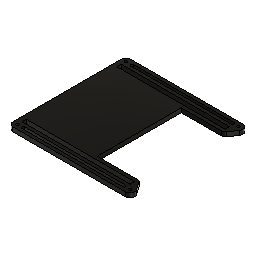
AssemblyCameraHolder v6 (Autodesk Fusion 360 archive; units mm, degrees)
design "CameraBase"
Autodesk Fusion 360 part; units mm, degrees
sketch "Sketch1" plane through (0, 0, 0) normal (0, 0, 1) x (1, 0, 0)
  line L0 (-62.5, 60.2) -> (62.5, 60.2) construction
  line L1 (62.5, 60.2) -> (62.5, -60.2) construction
  line L2 (62.5, -60.2) -> (-62.5, -60.2) construction
  line L3 (-62.5, -60.2) -> (-62.5, 60.2) construction
  line L4 (0, 0) -> (0, 60.2) construction
  line L5 (0, 0) -> (-62.5, 0) construction
  circle A0 centre (62.5, 60.2) radius 1.5
  circle A1 centre (-62.5, 60.2) radius 1.5
  circle A2 centre (62.5, -60.2) radius 1.5
  circle A3 centre (-62.5, -60.2) radius 1.5
  line L6 (-62.5, -65.2) -> (62.5, -65.2)
  line L7 (-67.5, -60.2) -> (-67.5, 60.2)
  line L8 (-62.5, 65.2) -> (62.5, 65.2)
  line L9 (-56, 61.7) -> (56, 61.7)
  line L10 (-56, 58.7) -> (56, 58.7)
  arc A4 (-56, 61.7) -> (-56, 58.7) centre (-56, 60.2) ccw
  arc A5 (56, 58.7) -> (56, 61.7) centre (56, 60.2) ccw
  arc A6 (-67.5, 60.2) -> (-62.5, 65.2) centre (-62.5, 60.2) ccw construction
  arc A7 (-62.5, 65.2) -> (-67.5, 60.2) centre (-62.5, 60.2) ccw
  line L11 (-62.5, 55.2) -> (57.5, 55.2)
  line L12 (57.5, 55.2) -> (57.5, 50.4)
  line L13 (57.5, 50.4) -> (-62.5, 50.4)
  line L14 (-62.5, 50.4) -> (-62.5, 55.2)
  line L15 (66.6668, 57.4363) -> (60.6251, 48.3272)
  arc A8 (62.5, 65.2) -> (66.6668, 57.4363) centre (62.5, 60.2) ccw construction
  arc A9 (66.6668, 57.4363) -> (62.5, 65.2) centre (62.5, 60.2) ccw
  arc A10 (60.6251, 48.3272) -> (60.6251, 48.3272) centre (57.5, 50.4) ccw construction
  line L16 (-56, -58.7) -> (56, -58.7)
  line L17 (-56, -61.7) -> (56, -61.7)
  arc A11 (-56, -58.7) -> (-56, -61.7) centre (-56, -60.2) ccw
  arc A12 (56, -61.7) -> (56, -58.7) centre (56, -60.2) ccw
  line L18 (-62.5, -55.2) -> (57.5, -55.2)
  line L19 (57.5, -55.2) -> (57.5, -50.4)
  line L20 (57.5, -50.4) -> (-62.5, -50.4)
  line L21 (-62.5, -50.4) -> (-62.5, -55.2)
  line L22 (57.5, -60.2) -> (57.5, -55.2) construction
  line L23 (60.6251, -48.3272) -> (66.6668, -57.4363)
  line L24 (57.5, -46.65) -> (12.5, -46.65)
  line L25 (12.5, 46.65) -> (12.5, -46.65)
  arc A13 (57.5, -46.65) -> (60.6251, -48.3272) centre (57.5, -50.4) ccw construction
  arc A14 (60.6251, -48.3272) -> (57.5, -46.65) centre (57.5, -50.4) ccw
  arc A15 (66.6668, -57.4363) -> (62.5, -65.2) centre (62.5, -60.2) ccw construction
  arc A16 (62.5, -65.2) -> (66.6668, -57.4363) centre (62.5, -60.2) ccw
  arc A17 (-62.5, -65.2) -> (-67.5, -60.2) centre (-62.5, -60.2) ccw construction
  arc A18 (-67.5, -60.2) -> (-62.5, -65.2) centre (-62.5, -60.2) ccw
  line L26 (57.5, -50.4) -> (57.5, 50.4) construction
  line L27 (57.5, 46.65) -> (12.5, 46.65)
  arc A19 (60.6251, 48.3272) -> (57.5, 46.65) centre (57.5, 50.4) ccw construction
  arc A20 (57.5, 46.65) -> (60.6251, 48.3272) centre (57.5, 50.4) ccw
  line L28 (57.5, 55.2) -> (57.5, 60.2) construction
  point P0 (-62.5, 0)
  point P1 (0, 60.2)
  dimension "d1" = 125
  dimension "d2" = 120.4
  dimension "d3" = 3
  dimension "d4" = 3
  dimension "d5" = 3
  dimension "d6" = 3
  dimension "d7" = 10
  dimension "d8" = 10
  dimension "d9" = 10
  dimension "d10" = 10
  dimension "d11" = 3
  dimension "d12" = 5
  dimension "d13" = 6.5
  dimension "d14" = 6.5
  dimension "d16" = 4.8
  dimension "d17" = 5
  dimension "d19" = 3
  dimension "d20" = 5
  dimension "d21" = 6.5
  dimension "d22" = 6.5
  dimension "d23" = 4.8
  dimension "d24" = 7.5
  dimension "d25" = 50
  dimension "d28" = 3.75
  constraint horizontal L0
  constraint vertical L1
  constraint horizontal L2
  constraint vertical L3
  constraint midpoint L3 P0
  constraint midpoint L0 P1
  constraint coincident L4.start L5.start
  constraint coincident P1 L4.end
  constraint coincident P0 L5.end
  constraint vertical L4
  constraint horizontal L5
  constraint coincident L0.end L1.start
  constraint coincident L0.start L3.end
  constraint coincident L1.end L2.start
  constraint coincident L2.end L3.start
  constraint concentric A1 A6
  constraint concentric A0 A8
  constraint concentric A2 A15
  constraint concentric A3 A17
  constraint tangent L6 A15
  constraint perpendicular L1 L6
  constraint tangent L7 A6
  constraint perpendicular L6 L7
  constraint tangent L8 A8
  constraint perpendicular L7 L8
  constraint parallel L8 L9
  constraint parallel L0 L10
  constraint tangent L10 A4
  constraint tangent L9 A4
  constraint tangent L10 A5
  constraint tangent L9 A5
  constraint concentric A6 A7
  constraint horizontal L11
  constraint vertical L12
  constraint horizontal L13
  constraint vertical L14
  constraint coincident L3 L11.start
  constraint coincident L12.end L13.start
  constraint tangent L15 A10
  constraint tangent L15 A8
  constraint perpendicular L2 L25
  constraint concentric A8 A9
  constraint perpendicular L3 L16
  constraint parallel L16 L17
  constraint tangent L16 A11
  constraint tangent L17 A11
  constraint tangent L16 A12
  constraint tangent L17 A12
  constraint horizontal L18
  constraint vertical L19
  constraint horizontal L20
  constraint vertical L21
  constraint coincident L3 L18.start
  constraint midpoint A12 L22.start
  constraint tangent L22 A15
  constraint coincident L19.end L20.start
  constraint tangent L23 A15
  constraint tangent L23 A13
  constraint tangent L24 A13
  constraint perpendicular L24 L25
  constraint concentric A13 A14
  constraint concentric A15 A16
  constraint coincident L18.start A17
  constraint concentric A17 A18
  constraint vertical L26
  constraint coincident L26 L27.start
  constraint tangent A10 L27
  constraint tangent L15 A19
  constraint concentric A19 A20
  constraint collinear L12 L26
  constraint midpoint A5 L28.end
  constraint collinear L12 L28
  measures "d1" distance of L0.start L0.end
  measures "d2" distance of L0.start L2.end
  measures "d3" diameter of A0
  measures "d4" diameter of A1
  measures "d5" diameter of A2
  measures "d6" diameter of A3
  measures "d7" diameter of A6
  measures "d8" diameter of A8
  measures "d9" diameter of A15
  measures "d10" diameter of A17
  measures "d11" distance of L9 L10
  measures "d12" distance of L8 A4.centre
  measures "d13" distance of L0.start A4.centre
  measures "d14" distance of L0.end A5.centre
  measures "d16" distance of L11.start L13.end
  measures "d17" distance of L0 L11
  measures "d19" distance of L16 L17
  measures "d20" distance of L6 A11.centre
  measures "d21" distance of L2.end A11.centre
  measures "d22" distance of L1.end A12.centre
  measures "d23" distance of L18.start L20.end
  measures "d24" diameter of A13
  measures "d25" distance of L1 L25
  measures "d28" radius of A19
extrude "Extrude1" add sketch "Sketch1" along normal blind 4.8

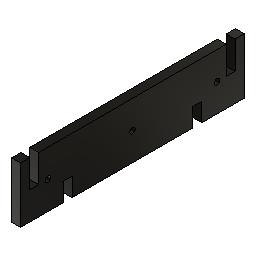
design "CameraHolder"
Autodesk Fusion 360 part; units mm, degrees
sketch "Sketch1" plane through (0, 0, 0) normal (1, 0, 0) x (0, 1, 0)
  line L0 (-60.2, 30) -> (-60.2, 0)
  line L1 (-60.2, 0) -> (-37.3, 0)
  line L2 (-37.3, 0) -> (-37.3, 10)
  line L3 (-37.3, 10) -> (-32.5, 10)
  line L4 (-32.5, 10) -> (-32.5, 0)
  line L5 (-32.5, 0) -> (32.5, 0)
  line L6 (32.5, 0) -> (32.5, 10)
  line L7 (32.5, 10) -> (37.3, 10)
  line L8 (37.3, 10) -> (37.3, 0)
  line L9 (37.3, 0) -> (60.2, 0)
  line L10 (60.2, 0) -> (60.2, 30)
  line L11 (60.2, 30) -> (55.2, 30)
  line L12 (55.2, 30) -> (55.2, 15)
  line L13 (55.2, 15) -> (50.4, 15)
  line L14 (50.4, 15) -> (50.4, 30)
  line L15 (50.4, 30) -> (-50.4, 30)
  line L16 (-50.4, 30) -> (-50.4, 15)
  line L17 (-50.4, 15) -> (-55.2, 15)
  line L18 (-55.2, 15) -> (-55.2, 30)
  line L19 (-55.2, 30) -> (-60.2, 30)
  line L20 (-55.2, 30) -> (-50.4, 30) construction
  line L21 (50.4, 30) -> (55.2, 30) construction
  line L22 (37.3, 0) -> (32.5, 0) construction
  line L23 (-32.5, 0) -> (-37.3, 0) construction
  line L24 (-50.4, 15) -> (50.4, 15) construction
  line L25 (0, 0) -> (0, 15) construction
  line L26 (0, 15) -> (0, 30) construction
  circle A0 centre (0, 15) radius 1.5
  circle A1 centre (-45.4, 15) radius 1.5
  circle A2 centre (45.4, 15) radius 1.5
  line L27 (-32.5, 10) -> (32.5, 10) construction
  point P0 (0, 15)
  point P1 (0, 15)
  point P2 (0, 30)
  dimension "d1" = 4.8
  dimension "d2" = 4.8
  dimension "d3" = 4.8
  dimension "d4" = 4.8
  dimension "d7" = 15
  dimension "d9" = 30
  dimension "d10" = 65
  dimension "d11" = 120.4
  dimension "d12" = 100.8
  dimension "d13" = 5
  dimension "d14" = 3
  dimension "d15" = 3
  dimension "d16" = 5
  dimension "d17" = 3
  dimension "d18" = 5
  dimension "d21" = 10
  constraint vertical L0
  constraint perpendicular L0 L1
  constraint perpendicular L1 L2
  constraint perpendicular L0 L3
  constraint perpendicular L1 L4
  constraint perpendicular L4 L5
  constraint perpendicular L3 L6
  constraint perpendicular L6 L7
  constraint perpendicular L7 L8
  constraint perpendicular L8 L9
  constraint perpendicular L9 L10
  constraint perpendicular L0 L11
  constraint perpendicular L11 L12
  constraint perpendicular L0 L13
  constraint perpendicular L13 L14
  constraint perpendicular L14 L15
  constraint perpendicular L15 L16
  constraint perpendicular L16 L17
  constraint perpendicular L15 L18
  constraint perpendicular L0 L19
  constraint perpendicular L18 L20
  constraint perpendicular L12 L21
  constraint perpendicular L6 L22
  constraint perpendicular L2 L23
  constraint perpendicular L14 L24
  constraint midpoint L24 P1
  constraint midpoint L5 L25.start
  constraint midpoint L15 P2
  constraint coincident L25.start origin
  constraint coincident P1 P0
  constraint coincident P2 L26.end
  constraint coincident L24 A1.centre
  constraint coincident L24 A2.centre
  constraint perpendicular L24 L25
  constraint perpendicular L6 L27
  measures "d1" distance of L2 L4
  measures "d2" distance of L6 L8
  measures "d3" distance of L12 L14
  measures "d4" distance of L16 L18
  measures "d7" distance of L15 L24
  measures "d9" distance of L0.start L0.end
  measures "d10" distance of L4 L6
  measures "d11" distance of L0 L10
  measures "d12" distance of L14 L16
  measures "d13" distance of L10 L12
  measures "d14" diameter of A0
  measures "d15" diameter of A1
  measures "d16" distance of L16 A1.centre
  measures "d17" diameter of A2
  measures "d18" distance of L14 A2.centre
  measures "d21" distance of L3 L5
extrude "Extrude1" add sketch "Sketch1" along normal blind 4.8

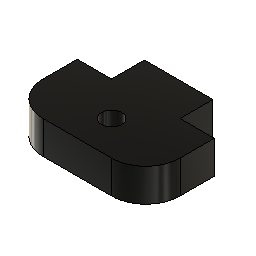
design "ThrowerLock"
Autodesk Fusion 360 part; units mm, degrees
sketch "Sketch1" plane through (0, 0, 0) normal (0, 0, 1) x (1, 0, 0)
  line L0 (-5, 9.8) -> (5, 9.8)
  line L1 (5, 9.8) -> (5, 5)
  line L2 (5, 5) -> (10, 5)
  line L3 (10, 5) -> (10, 0)
  line L4 (5, -5) -> (-5, -5)
  line L5 (-10, 0) -> (-10, 5)
  line L6 (-10, 5) -> (-5, 5)
  line L7 (-5, 5) -> (-5, 9.8)
  line L8 (0, 0) -> (0, 9.8) construction
  line L9 (0, 0) -> (10, 0) construction
  line L10 (0, 0) -> (0, -5) construction
  line L11 (-5, 5) -> (-5, 0) construction
  line L12 (0, 0) -> (-5, 0) construction
  circle A0 centre (0, 0) radius 1.5
  line L13 (-10, -5) -> (-10, 0) construction
  line L14 (-5, -5) -> (-10, -5) construction
  arc A1 (-5, -5) -> (-10, 0) centre (-5, 0) ccw construction
  arc A2 (-10, 0) -> (-5, -5) centre (-5, 0) ccw
  line L15 (10, -5) -> (5, -5) construction
  line L16 (10, 0) -> (10, -5) construction
  arc A3 (10, 0) -> (5, -5) centre (5, 0) ccw construction
  arc A4 (5, -5) -> (10, 0) centre (5, 0) ccw
  point P0 (0, 9.8)
  point P1 (0, -5)
  point P2 (5, 0)
  dimension "d1" = 10
  dimension "d2" = 5
  dimension "d3" = 4.8
  dimension "d5" = 3
  dimension "d6" = 10
  constraint horizontal L0
  constraint perpendicular L0 L1
  constraint perpendicular L1 L2
  constraint perpendicular L2 L3
  constraint perpendicular L1 L4
  constraint perpendicular L4 L5
  constraint perpendicular L5 L6
  constraint vertical L7
  constraint collinear L2 L6
  constraint midpoint L0 P0
  constraint coincident L8.start L9.start
  constraint coincident L0 P0
  constraint perpendicular L0 L8
  constraint coincident L3 L9.end
  constraint perpendicular L3 L9
  constraint coincident P0 L8.end
  constraint coincident L3.end L9.end
  constraint coincident L4 P1
  constraint perpendicular L4 L10
  constraint coincident P1 L10.end
  constraint perpendicular L6 L11
  constraint perpendicular L11 L12
  constraint coincident L11.end L12.end
  constraint tangent L4 A1
  constraint midpoint L9 P2
  constraint coincident P2 A3.centre
  constraint tangent L4 A3
  constraint perpendicular L4 L13
  constraint perpendicular L1 L14
  constraint tangent L14 A3
  constraint concentric A1 A2
  constraint perpendicular L1 L15
  constraint concentric A3 A4
  constraint parallel L3 L16
  constraint tangent L13 A2
  measures "d1" distance of L0.start L0.end
  measures "d2" distance of L1.end L2.end
  measures "d3" distance of L0.start L6.end
  measures "d5" diameter of A0
  measures "d6" distance of L4 L6
extrude "Extrude1" add sketch "Sketch1" along normal blind 4.8

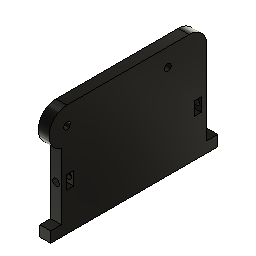
design "CameraHeadHolder"
Autodesk Fusion 360 part; units mm, degrees
sketch "Sketch1" plane through (0, 0, 0) normal (1, 0, 0) x (0, 1, 0)
  line L0 (-32.5, 4.8) -> (-37.3, 4.8)
  line L1 (-37.3, 4.8) -> (-37.3, 0)
  line L2 (-37.3, 0) -> (37.3, 0)
  line L3 (37.3, 0) -> (37.3, 4.8)
  line L4 (37.3, 4.8) -> (32.5, 4.8)
  line L5 (-32.5, 4.8) -> (-32.5, 34.2007)
  line L6 (-30, 49.8) -> (24.5, 49.8)
  line L7 (32.5, 41.8) -> (32.5, 4.8)
  line L8 (-30, 41.8) -> (15, 41.8) construction
  circle A0 centre (-30, 41.8) radius 1.5
  line L9 (15, 41.8) -> (24.5, 41.8) construction
  arc A1 (24.5, 49.8) -> (32.5, 41.8) centre (24.5, 41.8) ccw construction
  arc A2 (32.5, 41.8) -> (24.5, 49.8) centre (24.5, 41.8) ccw
  line L10 (24.5, 49.8) -> (32.5, 49.8) construction
  line L11 (32.5, 49.8) -> (32.5, 41.8) construction
  circle A3 centre (15, 41.8) radius 1.5
  circle A4 centre (-25, 41.8) radius 5 construction
  circle A5 centre (25, 41.8) radius 5 construction
  line L12 (-25, 41.8) -> (25, 41.8) construction
  line L13 (0, 41.8) -> (0, 0) construction
  arc A6 (-32.5, 34.2007) -> (-30, 49.8) centre (-30, 41.8) ccw construction
  arc A7 (-30, 49.8) -> (-32.5, 34.2007) centre (-30, 41.8) ccw
  point P0 (0, 41.8)
  dimension "d1" = 4.8
  dimension "d2" = 4.8
  dimension "d3" = 74.6
  dimension "d4" = 4.8
  dimension "d5" = 4.8
  dimension "d6" = 45
  dimension "d8" = 45
  dimension "d9" = 8
  dimension "d11" = 3
  dimension "d12" = 16
  dimension "d13" = 3
  dimension "d14" = 10
  dimension "d15" = 10
  dimension "d16" = 50
  dimension "d17" = 10
  constraint horizontal L0
  constraint perpendicular L0 L1
  constraint perpendicular L1 L2
  constraint perpendicular L2 L3
  constraint perpendicular L3 L4
  constraint midpoint L2 L13.end
  constraint coincident L13.end origin
  constraint perpendicular L0 L5
  constraint perpendicular L5 L6
  constraint perpendicular L4 L7
  constraint perpendicular L7 L8
  constraint tangent L7 A1
  constraint coincident L9.end A1.centre
  constraint parallel L8 L9
  constraint concentric A1 A2
  constraint perpendicular L5 L10
  constraint perpendicular L4 L11
  constraint coincident L8.end L9.start
  constraint coincident L8 A4.centre
  constraint coincident L9 A5.centre
  constraint coincident A4.centre L12.start
  constraint coincident A5.centre L12.end
  constraint midpoint L12 P0
  constraint coincident P0 L13.start
  constraint vertical L13
  constraint coincident L8.start A0.centre
  constraint tangent L6 A6
  constraint concentric A6 A7
  constraint concentric A0 A7
  measures "d1" distance of L0.start L0.end
  measures "d2" distance of L0.end L1.end
  measures "d3" distance of L1.end L2.end
  measures "d4" distance of L2.end L3.end
  measures "d5" distance of L3.end L4.end
  measures "d6" distance of L4 L6
  measures "d8" distance of L8.start L8.end
  measures "d9" distance of L6 L8
  measures "d11" diameter of A0
  measures "d12" diameter of A1
  measures "d13" diameter of A3
  measures "d14" diameter of A4
  measures "d15" diameter of A5 L6
  measures "d16" distance of A4.centre A5.centre
  measures "d17" distance of L8.end A5.centre
extrude "Extrude1" add sketch "Sketch1" along normal blind 4.8
sketch "Sketch2" plane through (0, -32.5, 0) normal (0, -1, 0) x (1, 0, 0)
  line L0 (0, 34.2007) -> (0, 4.8)
  line L1 (0, 4.8) -> (4.8, 4.8)
  line L2 (4.8, 4.8) -> (4.8, 34.2007)
  line L3 (4.8, 34.2007) -> (0, 34.2007)
  line L4 (0, 4.8) -> (0, 0)
  line L5 (0, 0) -> (4.8, 0)
  line L6 (4.8, 0) -> (4.8, 4.8)
  line L7 (4.8, 4.8) -> (0, 4.8)
  circle A0 centre (2.4, 20) radius 1.5
  dimension "d20" = 3
  dimension "d21" = 20
  dimension "d22" = 2.4
  measures "d20" diameter of A0
  measures "d21" distance of L5 A0.centre
  measures "d22" distance of L2 A0.centre
hole "Hole1" at (2.4, -32.5, 20) direction (0, 1, 0) diameter 3 depth 7.2 tip angle 118
sketch "Sketch3" plane through (0, 32.5, 0) normal (0, 1, 0) x (-1, 0, 0)
  line L0 (0, 4.8) -> (0, 41.8)
  line L1 (0, 41.8) -> (-4.8, 41.8)
  line L2 (-4.8, 41.8) -> (-4.8, 4.8)
  line L3 (-4.8, 4.8) -> (0, 4.8)
  line L4 (0, 0) -> (0, 4.8)
  line L5 (0, 4.8) -> (-4.8, 4.8)
  line L6 (-4.8, 4.8) -> (-4.8, 0)
  line L7 (-4.8, 0) -> (0, 0)
  circle A0 centre (-2.4, 20) radius 1.5
  dimension "d26" = 3
  dimension "d27" = 20
  dimension "d28" = 2.4
  measures "d26" diameter of A0
  measures "d27" distance of L7 A0.centre
  measures "d28" distance of L0 A0.centre
hole "Hole2" at (2.4, 32.5, 20) direction (0, -1, 0) diameter 3 depth 7.2 tip angle 118
sketch "Sketch4" plane through (4.8, 0, 0) normal (1, 0, 0) x (0, 1, 0)
  circle A0 centre (15, 41.8) radius 1.5
  circle A1 centre (-30, 41.8) radius 1.5
  arc A2 (32.5, 41.8) -> (24.5, 49.8) centre (24.5, 41.8) ccw
  line L0 (24.5, 49.8) -> (-30, 49.8)
  arc A3 (-30, 49.8) -> (-32.5, 34.2007) centre (-30, 41.8) ccw
  line L1 (-32.5, 34.2007) -> (-32.5, 4.8)
  line L2 (-32.5, 4.8) -> (-37.3, 4.8)
  line L3 (-37.3, 4.8) -> (-37.3, 0)
  line L4 (-37.3, 0) -> (37.3, 0)
  line L5 (37.3, 0) -> (37.3, 4.8)
  line L6 (37.3, 4.8) -> (32.5, 4.8)
  line L7 (32.5, 4.8) -> (32.5, 41.8)
  line L8 (-32.5, 18.5) -> (-25.3, 18.5) construction
  line L9 (-25.3, 18.5) -> (-25.3, 21.5) construction
  line L10 (-25.3, 21.5) -> (-32.5, 21.5) construction
  line L11 (32.5, 21.5) -> (25.3, 21.5) construction
  line L12 (25.3, 21.5) -> (25.3, 18.5) construction
  line L13 (25.3, 18.5) -> (32.5, 18.5) construction
  line L14 (-25.3, 20) -> (25.3, 20) construction
  line L15 (-30, 17) -> (-27, 17)
  line L16 (-27, 17) -> (-27, 23)
  line L17 (-27, 23) -> (-30, 23)
  line L18 (-30, 23) -> (-30, 17)
  line L19 (-25.3, 20) -> (-27, 20) construction
  line L20 (27, 23) -> (30, 23)
  line L21 (30, 23) -> (30, 17)
  line L22 (30, 17) -> (27, 17)
  line L23 (27, 17) -> (27, 23)
  line L24 (27, 20) -> (25.3, 20) construction
  point P0 (-25.3, 20)
  point P1 (25.3, 20)
  point P2 (-27, 20)
  point P3 (27, 20)
  dimension "d32" = 7.2
  dimension "d33" = 3
  dimension "d34" = 7.2
  dimension "d35" = 3
  dimension "d36" = 20
  dimension "d37" = 3
  dimension "d38" = 6
  dimension "d39" = 2.5
  dimension "d40" = 3
  dimension "d41" = 6
  dimension "d42" = 2.5
  constraint coincident L1 L8.start
  constraint perpendicular L1 L8
  constraint perpendicular L8 L9
  constraint coincident L1 L10.end
  constraint perpendicular L1 L10
  constraint midpoint L9 P0
  constraint coincident L7 L11.start
  constraint perpendicular L7 L11
  constraint perpendicular L11 L12
  constraint coincident L7 L13.end
  constraint perpendicular L7 L13
  constraint midpoint L12 P1
  constraint coincident P0 L14.start
  constraint coincident P1 L14.end
  constraint horizontal L14
  constraint horizontal L15
  constraint vertical L16
  constraint horizontal L17
  constraint vertical L18
  constraint midpoint L16 P2
  constraint coincident P2 L19.end
  constraint horizontal L19
  constraint horizontal L20
  constraint vertical L21
  constraint horizontal L22
  constraint vertical L23
  constraint midpoint L23 P3
  constraint coincident P3 L24.start
  constraint horizontal L24
  measures "d32" distance of L8.start L8.end
  measures "d33" distance of L8.end L9.end
  measures "d34" distance of L11.start L11.end
  measures "d35" distance of L11.end L12.end
  measures "d36" distance of L4 L14
  measures "d37" distance of L15.start L15.end
  measures "d38" distance of L15.start L17.end
  measures "d39" distance of L1 L18
  measures "d40" distance of L20.start L20.end
  measures "d41" distance of L20.start L22.end
  measures "d42" distance of L7 L21
extrude "Extrude2" cut sketch "Sketch4" against normal through all contours L15 L16 L17 L18 | L20 L21 L22 L23

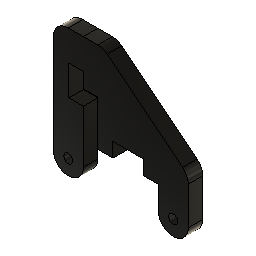
design "CameraHolderSide"
Autodesk Fusion 360 part; units mm, degrees
sketch "Sketch1" plane through (0, 0, 0) normal (0, 1, 0) x (1, 0, 0)
  line L0 (-4.8, 0) -> (-4.8, -10)
  line L1 (0, 0) -> (0, -15)
  line L2 (0, -15) -> (-4.8, -15)
  line L3 (0, 0) -> (-4.8, 0) construction
  line L4 (-4.8, 0) -> (-4.8, 7.5)
  line L5 (0, -30) -> (-4.8, -30)
  line L6 (0, -15) -> (0, -30) construction
  line L7 (-4.8, -15) -> (-4.8, -30) construction
  line L8 (-4.8, -30) -> (-9.8, -30)
  line L9 (-14.8, 7.5) -> (-14.8, -25)
  arc A0 (-9.8, -30) -> (-14.8, -25) centre (-9.8, -25) ccw construction
  arc A1 (-14.8, -25) -> (-9.8, -30) centre (-9.8, -25) ccw
  arc A2 (-14.8, 7.5) -> (-4.8, 7.5) centre (-9.8, 7.5) ccw construction
  arc A3 (-4.8, 7.5) -> (-14.8, 7.5) centre (-9.8, 7.5) ccw
  circle A4 centre (-9.8, 7.5) radius 1.5
  line L10 (0, 0) -> (5, 0)
  line L11 (5, 0) -> (5, -4.8)
  line L12 (5, -4.8) -> (15, -4.8)
  line L13 (15, -4.8) -> (15, 0)
  line L14 (15, 0) -> (20, 0)
  line L15 (20, 0) -> (20, 7.5)
  line L16 (30, 7.5) -> (30, -5)
  line L17 (3.1235, -28.9043) -> (28.1235, -8.9043)
  arc A5 (3.1235, -28.9043) -> (0, -30) centre (0, -25) ccw construction
  arc A6 (0, -30) -> (3.1235, -28.9043) centre (0, -25) ccw
  arc A7 (30, -5) -> (28.1235, -8.9043) centre (25, -5) ccw construction
  arc A8 (28.1235, -8.9043) -> (30, -5) centre (25, -5) ccw
  arc A9 (20, 7.5) -> (30, 7.5) centre (25, 7.5) ccw construction
  arc A10 (30, 7.5) -> (20, 7.5) centre (25, 7.5) ccw
  circle A11 centre (25, 7.5) radius 1.5
  line L18 (-4.8, -10) -> (-9.6, -10)
  line L19 (-9.6, -10) -> (-9.6, -20)
  line L20 (-9.6, -20) -> (-4.8, -20)
  line L21 (-4.8, -20) -> (-4.8, -15)
  line L22 (-9.8, 7.5) -> (-9.8, -25) construction
  line L23 (-4.8, 7.5) -> (20, 7.5) construction
  dimension "d1" = 15
  dimension "d3" = 4.8
  dimension "d4" = 7.5
  dimension "d5" = 4.8
  dimension "d6" = 15
  dimension "d7" = 10
  dimension "d8" = 10
  dimension "d9" = 3
  dimension "d10" = 5
  dimension "d11" = 4.8
  dimension "d12" = 10
  dimension "d13" = 4.8
  dimension "d14" = 5
  dimension "d16" = 10
  dimension "d17" = 10
  dimension "d18" = 5
  dimension "d19" = 5
  dimension "d20" = 5
  dimension "d21" = 3
  dimension "d22" = 4.8
  dimension "d23" = 10
  dimension "d24" = 5
  constraint vertical L0
  constraint coincident L1.start L3.start
  constraint vertical L1
  constraint perpendicular L0 L2
  constraint perpendicular L0 L3
  constraint perpendicular L3 L4
  constraint parallel L2 L5
  constraint perpendicular L5 L6
  constraint tangent L7 A0
  constraint tangent L8 A0
  constraint tangent L4 A2
  constraint tangent L9 A0
  constraint vertical L9
  constraint concentric A0 A1
  constraint concentric A2 A3
  constraint concentric A3 A4
  constraint collinear L5 L8
  constraint perpendicular L1 L10
  constraint perpendicular L10 L11
  constraint perpendicular L11 L12
  constraint perpendicular L12 L13
  constraint perpendicular L13 L14
  constraint perpendicular L14 L15
  constraint tangent L15 A9
  constraint coincident L6 A5.centre
  constraint tangent L16 A7
  constraint tangent L17 A7
  constraint tangent L17 A5
  constraint concentric A5 A6
  constraint concentric A7 A8
  constraint concentric A9 A10
  constraint tangent L16 A9
  constraint concentric A10 A11
  constraint perpendicular L0 L18
  constraint perpendicular L18 L19
  constraint coincident L7 L20.end
  constraint perpendicular L7 L20
  constraint perpendicular L2 L21
  constraint coincident A2.centre A3.centre
  constraint coincident A0.centre A1.centre
  constraint perpendicular L3 L22
  constraint perpendicular L15 L23
  measures "d1" distance of L0.start L2.end
  measures "d3" distance of L2.end L1.end
  measures "d4" distance of L0.start L4.end
  measures "d5" distance of L5.start L5.end
  measures "d6" distance of L2 L5
  measures "d7" diameter of A0
  measures "d8" diameter of A2
  measures "d9" diameter of A4
  measures "d10" distance of L1.start L10.end
  measures "d11" distance of L10.end L11.end
  measures "d12" distance of L11.end L12.end
  measures "d13" distance of L12.end L13.end
  measures "d14" distance of L13.end L14.end
  measures "d16" diameter of A9
  measures "d17" diameter of A7
  measures "d18" distance of L14 A7.centre
  measures "d19" radius of A5
  measures "d20" distance of L15 A7.centre
  measures "d21" diameter of A11
  measures "d22" distance of L0.end L18.end
  measures "d23" distance of L18.end L19.end
  measures "d24" distance of L2 L18
extrude "Extrude1" add sketch "Sketch1" along normal blind 4.8

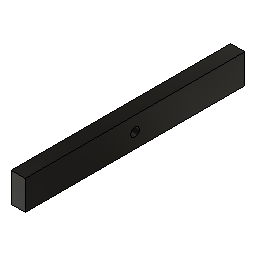
design "CameraLevelLock"
Autodesk Fusion 360 part; units mm, degrees
sketch "Sketch1" plane through (0, 0, 0) normal (1, 0, 0) x (0, 1, 0)
  line L0 (-37.3, 5) -> (37.3, 5)
  line L1 (37.3, 5) -> (37.3, -5)
  line L2 (37.3, -5) -> (-37.3, -5)
  line L3 (-37.3, -5) -> (-37.3, 5)
  line L4 (0, 0) -> (0, 5) construction
  line L5 (0, 0) -> (-37.3, 0) construction
  circle A0 centre (0, 0) radius 1.5
  point P0 (0, 5)
  point P1 (-37.3, 0)
  dimension "d1" = 3
  dimension "d2" = 10
  dimension "d3" = 74.6
  constraint horizontal L0
  constraint vertical L1
  constraint horizontal L2
  constraint vertical L3
  constraint midpoint L0 P0
  constraint midpoint L3 P1
  constraint coincident L4.start L5.start
  constraint coincident P0 L4.end
  constraint coincident P1 L5.end
  constraint horizontal L5
  constraint vertical L4
  measures "d1" diameter of A0
  measures "d2" distance of L0.start L2.end
  measures "d3" distance of L0.start L0.end
extrude "Extrude1" add sketch "Sketch1" along normal blind 4.8

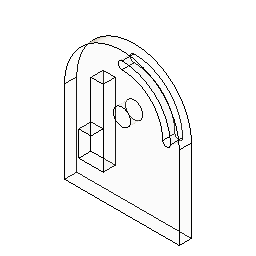
design "CameraLevel"
Autodesk Fusion 360 part; units mm, degrees
sketch "Sketch1" plane through (0, 0, 0) normal (0, 1, 0) x (1, 0, 0)
  line L0 (0, 0) -> (-4.8, 0)
  line L1 (-4.8, 0) -> (-4.8, -10)
  line L2 (-4.8, -10) -> (0, -10)
  line L3 (0, -10) -> (0, -30)
  line L4 (0, -30) -> (4.8, -30)
  line L5 (4.8, -30) -> (4.8, 0)
  line L6 (4.8, 0) -> (0, 0)
  line L7 (0, 0) -> (0, -10) construction
  line L8 (-10.4, 10) -> (34.8, 10)
  line L9 (9.8, -25) -> (14.6, -25) construction
  line L10 (14.6, -25) -> (14.6, -20.2) construction
  line L11 (14.6, -20.2) -> (9.8, -20.2) construction
  line L12 (9.8, -20.2) -> (9.8, -25) construction
  line L13 (9.8, -22.6) -> (29.8, -22.6) construction
  line L14 (12.2, -20.2) -> (12.2, -40.2) construction
  circle A0 centre (12.2, -22.6) radius 3.3941
  arc A1 (31.3, -22.6) -> (12.2, -41.7) centre (12.2, -22.6) ccw construction
  arc A2 (12.2, -41.7) -> (31.3, -22.6) centre (12.2, -22.6) ccw
  arc A3 (28.3, -22.6) -> (12.2, -38.7) centre (12.2, -22.6) ccw construction
  arc A4 (12.2, -38.7) -> (28.3, -22.6) centre (12.2, -22.6) ccw
  arc A5 (12.2, -38.7) -> (12.2, -41.7) centre (12.2, -40.2) ccw
  arc A6 (12.2, -41.7) -> (12.2, -38.7) centre (12.2, -40.2) ccw construction
  arc A7 (31.3, -22.6) -> (28.3, -22.6) centre (29.8, -22.6) ccw
  arc A8 (28.3, -22.6) -> (31.3, -22.6) centre (29.8, -22.6) ccw construction
  circle A9 centre (12.2, -40.2) radius 5 construction
  line L15 (-10.4, 10) -> (-10.4, -22.6)
  arc A10 (12.2, -45.2) -> (12.2, -45.2) centre (12.2, -22.6) ccw
  line L16 (34.8, -22.6) -> (34.8, 10)
  line L17 (9.8, -25) -> (4.8, -25) construction
  arc A11 (34.8, -22.6) -> (-10.4, -22.6) centre (12.2, -22.6) ccw construction
  arc A12 (-10.4, -22.6) -> (12.2, -45.2) centre (12.2, -22.6) ccw
  arc A13 (12.2, -45.2) -> (34.8, -22.6) centre (12.2, -22.6) ccw
  point P0 (12.2, -20.2)
  point P1 (9.8, -22.6)
  point P2 (12.2, -22.6)
  dimension "d23" = 4.8
  dimension "d24" = 10
  dimension "d26" = 4.8
  dimension "d27" = 10
  dimension "d31" = 4.8
  dimension "d32" = 4.8
  dimension "d33" = 20
  dimension "d34" = 20
  dimension "d35" = 3
  dimension "d36" = 3
  dimension "d37" = 10
  dimension "d38" = 30
  dimension "d40" = 5
  dimension "d41" = 5
  constraint perpendicular L0 L1
  constraint perpendicular L1 L2
  constraint perpendicular L2 L3
  constraint perpendicular L3 L4
  constraint perpendicular L4 L5
  constraint coincident L0.start L6.end
  constraint perpendicular L2 L7
  constraint parallel L6 L8
  constraint horizontal L9
  constraint vertical L10
  constraint horizontal L11
  constraint vertical L12
  constraint midpoint L11 P0
  constraint midpoint L12 P1
  constraint coincident P1 L13.start
  constraint perpendicular L12 L13
  constraint coincident P0 L14.start
  constraint perpendicular L11 L14
  constraint coincident L13 P2
  constraint coincident L14 P2
  constraint coincident L14.end A5.centre
  constraint coincident L13.end A7.centre
  constraint coincident P2 A0.centre
  constraint coincident L10.end A0
  constraint tangent A3 A7
  constraint concentric A0 A1
  constraint tangent A1 A7
  constraint concentric A1 A2
  constraint coincident L14 A3.end
  constraint coincident L13 A3.start
  constraint concentric A3 A4
  constraint concentric A5 A6
  constraint concentric A7 A8
  constraint concentric A5 A9
  constraint coincident A9 A10.start
  constraint tangent A10 L16
  constraint perpendicular L8 L16
  constraint vertical L15
  constraint collinear L0 L6
  constraint perpendicular L8 L15
  constraint perpendicular L5 L17
  constraint coincident L5 L17.end
  constraint tangent A9 A10
  constraint coincident A10 L16.start
  constraint concentric A0 A11
  constraint tangent A9 A11
  constraint tangent L16 A11
  constraint tangent L15 A11
  constraint concentric A11 A12
  constraint concentric A11 A13
  measures "d23" distance of L0.start L0.end
  measures "d24" distance of L0.end L1.end
  measures "d26" distance of L3.end L4.end
  measures "d27" distance of L6 L8
  measures "d31" distance of L9.start L9.end
  measures "d32" distance of L9.start L11.end
  measures "d33" distance of P1 L13.end
  measures "d34" distance of P0 L14.end
  measures "d35" diameter of A5
  measures "d36" diameter of A7
  measures "d37" diameter of A9
  measures "d38" distance of L4 L6
  measures "d40" distance of L9.start L17.end
  measures "d41" distance of L4 L17
extrude "Extrude1" add sketch "Sketch1" along normal blind 4.8 contours L0 L1 L5 L6 L8 L15 A10 L16 | L1 L2 L3 L4 L5 A10 A12 A13
